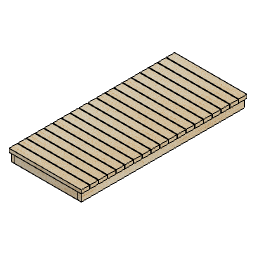
model (Autodesk Fusion 360 design; units mm, degrees)
Autodesk Fusion 360 part; units mm, degrees
sketch "Sketch1" plane through (0, 0, 0) normal (0, 0, 1) x (1, 0, 0) in component "base"
  line L0 (0, 0) -> (762, 0)
  line L1 (762, 0) -> (762, 1778)
  line L2 (762, 1778) -> (0, 1778)
  line L3 (0, 1778) -> (0, 0)
  line L4 (38.1, 38.1) -> (723.9, 38.1)
  line L5 (723.9, 38.1) -> (723.9, 1739.9)
  line L6 (723.9, 1739.9) -> (38.1, 1739.9)
  line L7 (38.1, 1739.9) -> (38.1, 38.1)
  line L8 (38.1, 1739.9) -> (38.1, 1778)
  line L9 (723.9, 1739.9) -> (723.9, 1778)
  line L10 (723.9, 38.1) -> (723.9, 0)
  line L11 (38.1, 38.1) -> (38.1, 0)
  line L12 (400.05, 1739.9) -> (361.95, 1739.9)
  line L13 (361.95, 1739.9) -> (361.95, 38.1)
  line L14 (361.95, 38.1) -> (400.05, 38.1)
  line L15 (400.05, 38.1) -> (400.05, 1739.9)
  line L16 (361.95, 889) -> (38.1, 889) construction
  line L17 (400.05, 889) -> (723.9, 889) construction
  line L18 (400.05, 1391.92) -> (723.9, 1391.92)
  line L19 (723.9, 1391.92) -> (723.9, 1430.02)
  line L20 (723.9, 1430.02) -> (400.05, 1430.02)
  line L21 (400.05, 1430.02) -> (400.05, 1391.92)
  line L22 (38.1, 386.08) -> (361.95, 386.08)
  line L23 (361.95, 386.08) -> (361.95, 347.98)
  line L24 (361.95, 347.98) -> (38.1, 347.98)
  line L25 (38.1, 347.98) -> (38.1, 386.08)
  line L26 (38.1, 1082.04) -> (361.95, 1082.04)
  line L27 (361.95, 1082.04) -> (361.95, 1043.94)
  line L28 (361.95, 1043.94) -> (38.1, 1043.94)
  line L29 (38.1, 1043.94) -> (38.1, 1082.04)
  line L30 (400.05, 734.06) -> (723.9, 734.06)
  line L31 (723.9, 734.06) -> (723.9, 695.96)
  line L32 (723.9, 695.96) -> (400.05, 695.96)
  line L33 (400.05, 695.96) -> (400.05, 734.06)
  line L34 (561.975, 734.06) -> (561.975, 889) construction
  line L35 (200.025, 386.08) -> (561.975, 695.96) construction
  line L36 (561.975, 734.06) -> (200.025, 1043.94) construction
  line L37 (561.975, 695.96) -> (561.975, 38.1) construction
  line L38 (200.025, 347.98) -> (561.975, 38.1) construction
  line L39 (200.025, 1082.04) -> (561.975, 1391.92) construction
  line L40 (200.025, 1082.04) -> (200.025, 1739.9) construction
  line L41 (561.975, 1430.02) -> (200.025, 1739.9) construction
  dimension "d3" = 1778
  dimension "d4" = 762
  dimension "d5" = -38.1
  dimension "d6" = 38.1
  dimension "d7" = 38.1
  dimension "d8" = 38.1
  dimension "d9" = 38.1
  dimension "d10" = 38.1
  constraint horizontal L0
  constraint vertical L1
  constraint horizontal L2
  constraint vertical L3
  constraint coincident L0.start L3.end
  constraint coincident L2 L8.end
  constraint perpendicular L2 L8
  constraint coincident L2 L9.end
  constraint perpendicular L2 L9
  constraint coincident L0 L10.end
  constraint perpendicular L0 L10
  constraint coincident L0 L11.end
  constraint perpendicular L0 L11
  constraint horizontal L12
  constraint vertical L13
  constraint horizontal L14
  constraint vertical L15
  constraint coincident L4 L13.end
  constraint coincident L6 L12.start
  constraint midpoint L13 L16.start
  constraint midpoint L7 L16.end
  constraint midpoint L15 L17.start
  constraint midpoint L5 L17.end
  constraint equal L16 L17
  constraint horizontal L18
  constraint vertical L19
  constraint horizontal L20
  constraint vertical L21
  constraint coincident L5 L19.end
  constraint coincident L15 L18.start
  constraint horizontal L22
  constraint vertical L23
  constraint horizontal L24
  constraint vertical L25
  constraint coincident L13 L23.end
  constraint coincident L7 L22.start
  constraint midpoint L24 L38.start
  constraint horizontal L26
  constraint vertical L27
  constraint horizontal L28
  constraint vertical L29
  constraint coincident L13 L27.end
  constraint coincident L7 L26.start
  constraint horizontal L30
  constraint vertical L31
  constraint horizontal L32
  constraint vertical L33
  constraint coincident L5 L31.end
  constraint coincident L15 L30.start
  constraint midpoint L28 L36.end
  constraint midpoint L30 L34.start
  constraint midpoint L17 L34.end
  constraint perpendicular L17 L34
  constraint midpoint L22 L35.start
  constraint midpoint L32 L35.end
  constraint equal L35 L36
  constraint coincident L4 L37.end
  constraint perpendicular L4 L37
  constraint equal L35 L38
  constraint midpoint L26 L39.start
  constraint midpoint L18 L39.end
  constraint coincident L6 L40.end
  constraint perpendicular L6 L40
  constraint equal L36 L39
  constraint midpoint L20 L41.start
  constraint equal L39 L41
  measures "d3" distance of L0.start L2.end
  measures "d4" distance of L0.start L0.end
  measures "d6" distance of L13.end L14.end
  measures "d7" distance of L22.start L24.end
  measures "d8" distance of L18.end L19.end
  measures "d9" distance of L30.end L31.end
  measures "d10" distance of L26.start L28.end
extrude "Extrude1" add sketch "Sketch1" along normal blind 88.9 contours L0 L4 L10 L11 L14 | L2 L6 L8 L9 L12 | L7 L13 L22 L23 L24 L25 | L5 L15 L30 L31 L32 L33 | L7 L13 L26 L27 L28 L29 | L5 L15 L18 L19 L20 L21 makes body 1 at (146.05, 1082.04, 29.6333) makes body 2 at (266.7, 38.1, 29.6333) makes body 3 at (508, 1391.92, 29.6333) makes body 4 at (615.95, 695.96, 29.6333) makes body 5 at (146.05, 386.08, 29.6333) makes body 6 at (495.3, 1778, 29.6333) in component "base"
extrude "Extrude2" add sketch "Sketch1" along normal blind 88.9 separate body contours L0 L2 L3 L7 L8 L11 L25 L29 | L0 L1 L2 L5 L9 L10 L19 L31 | L4 L6 L12 L13 L14 L15 L21 L23 L27 L33 makes body 7 at (361.95, 1172.6333, 29.6333) makes body 8 at (723.9, 1185.3333, 29.6333) makes body 9 at (38.1, 592.6667, 29.6333) in component "base"
sketch "Sketch1 (2)" plane through (0, 0, 88.9) normal (0, 0, 1) x (-1, 0, 0) in component "decking"
  line L0 (-38.1, 0) -> (-38.1, -1778)
  line L1 (-38.1, -1778) -> (0, -1778)
  line L2 (0, -1778) -> (0, 0)
  line L3 (0, 0) -> (-38.1, 0)
  line L4 (12.7, -1790.7) -> (-774.7, -1790.7)
  line L5 (-774.7, -1790.7) -> (-774.7, -1701.8)
  line L6 (-774.7, -1701.8) -> (12.7, -1701.8)
  line L7 (12.7, -1701.8) -> (12.7, -1790.7)
  line L8 (12.7, -1695.45) -> (-774.7, -1695.45)
  line L9 (-774.7, -1695.45) -> (-774.7, -1606.55)
  line L10 (-774.7, -1606.55) -> (12.7, -1606.55)
  line L11 (12.7, -1606.55) -> (12.7, -1695.45)
  line L12 (12.7, -1600.2) -> (-774.7, -1600.2)
  line L13 (-774.7, -1600.2) -> (-774.7, -1511.3)
  line L14 (-774.7, -1511.3) -> (12.7, -1511.3)
  line L15 (12.7, -1511.3) -> (12.7, -1600.2)
  line L16 (12.7, -1504.95) -> (-774.7, -1504.95)
  line L17 (-774.7, -1504.95) -> (-774.7, -1416.05)
  line L18 (-774.7, -1416.05) -> (12.7, -1416.05)
  line L19 (12.7, -1416.05) -> (12.7, -1504.95)
  line L20 (12.7, -1409.7) -> (-774.7, -1409.7)
  line L21 (-774.7, -1409.7) -> (-774.7, -1320.8)
  line L22 (-774.7, -1320.8) -> (12.7, -1320.8)
  line L23 (12.7, -1320.8) -> (12.7, -1409.7)
  line L24 (12.7, -1314.45) -> (-774.7, -1314.45)
  line L25 (-774.7, -1314.45) -> (-774.7, -1225.55)
  line L26 (-774.7, -1225.55) -> (12.7, -1225.55)
  line L27 (12.7, -1225.55) -> (12.7, -1314.45)
  line L28 (12.7, -1219.2) -> (-774.7, -1219.2)
  line L29 (-774.7, -1219.2) -> (-774.7, -1130.3)
  line L30 (-774.7, -1130.3) -> (12.7, -1130.3)
  line L31 (12.7, -1130.3) -> (12.7, -1219.2)
  line L32 (12.7, -1123.95) -> (-774.7, -1123.95)
  line L33 (-774.7, -1123.95) -> (-774.7, -1035.05)
  line L34 (-774.7, -1035.05) -> (12.7, -1035.05)
  line L35 (12.7, -1035.05) -> (12.7, -1123.95)
  line L36 (12.7, -1028.7) -> (-774.7, -1028.7)
  line L37 (-774.7, -1028.7) -> (-774.7, -939.8)
  line L38 (-774.7, -939.8) -> (12.7, -939.8)
  line L39 (12.7, -939.8) -> (12.7, -1028.7)
  line L40 (12.7, -933.45) -> (-774.7, -933.45)
  line L41 (-774.7, -933.45) -> (-774.7, -844.55)
  line L42 (-774.7, -844.55) -> (12.7, -844.55)
  line L43 (12.7, -844.55) -> (12.7, -933.45)
  line L44 (12.7, -838.2) -> (-774.7, -838.2)
  line L45 (-774.7, -838.2) -> (-774.7, -749.3)
  line L46 (-774.7, -749.3) -> (12.7, -749.3)
  line L47 (12.7, -749.3) -> (12.7, -838.2)
  line L48 (12.7, -742.95) -> (-774.7, -742.95)
  line L49 (-774.7, -742.95) -> (-774.7, -654.05)
  line L50 (-774.7, -654.05) -> (12.7, -654.05)
  line L51 (12.7, -654.05) -> (12.7, -742.95)
  line L52 (12.7, -647.7) -> (-774.7, -647.7)
  line L53 (-774.7, -647.7) -> (-774.7, -558.8)
  line L54 (-774.7, -558.8) -> (12.7, -558.8)
  line L55 (12.7, -558.8) -> (12.7, -647.7)
  line L56 (12.7, -552.45) -> (-774.7, -552.45)
  line L57 (-774.7, -552.45) -> (-774.7, -463.55)
  line L58 (-774.7, -463.55) -> (12.7, -463.55)
  line L59 (12.7, -463.55) -> (12.7, -552.45)
  line L60 (12.7, -457.2) -> (-774.7, -457.2)
  line L61 (-774.7, -457.2) -> (-774.7, -368.3)
  line L62 (-774.7, -368.3) -> (12.7, -368.3)
  line L63 (12.7, -368.3) -> (12.7, -457.2)
  line L64 (12.7, -361.95) -> (-774.7, -361.95)
  line L65 (-774.7, -361.95) -> (-774.7, -273.05)
  line L66 (-774.7, -273.05) -> (12.7, -273.05)
  line L67 (12.7, -273.05) -> (12.7, -361.95)
  line L68 (12.7, -266.7) -> (-774.7, -266.7)
  line L69 (-774.7, -266.7) -> (-774.7, -177.8)
  line L70 (-774.7, -177.8) -> (12.7, -177.8)
  line L71 (12.7, -177.8) -> (12.7, -266.7)
  line L72 (12.7, -171.45) -> (-774.7, -171.45)
  line L73 (-774.7, -171.45) -> (-774.7, -82.55)
  line L74 (-774.7, -82.55) -> (12.7, -82.55)
  line L75 (12.7, -82.55) -> (12.7, -171.45)
  line L76 (12.7, -76.2) -> (-774.7, -76.2)
  line L77 (-774.7, -76.2) -> (-774.7, 12.7)
  line L78 (-774.7, 12.7) -> (12.7, 12.7)
  line L79 (12.7, 12.7) -> (12.7, -76.2)
  line L80 (0, -1778) -> (12.7, -1778) construction
  line L81 (-774.7, -1778) -> (-762, -1778) construction
  line L82 (-723.9, -1778) -> (-38.1, -1778) construction
  line L83 (-381, -1778) -> (-381, -1790.7) construction
  point P0 (-762, -1778)
  dimension "d15" = 787.4
  dimension "d16" = 88.9
  dimension "d19" = 0
  dimension "d20" = 95.25
  constraint horizontal L4
  constraint vertical L5
  constraint horizontal L6
  constraint vertical L7
  constraint coincident L1.end L2.start
  constraint coincident L7 L80.end
  constraint perpendicular L7 L80
  constraint coincident L5 L81.start
  constraint coincident P0 L81.end
  constraint perpendicular L5 L81
  constraint equal L80 L81
  constraint midpoint L82 L83.start
  constraint midpoint L4 L83.end
  constraint equal L80 L83
  measures "d15" distance of L4.start L4.end
  measures "d16" distance of L4.end L5.end
extrude "Extrude1'" add sketch "Sketch1 (2)" along normal blind 38.1 separate body contours L0 L2 L3 L76 | L0 L2 L3 L76 L77 L78 L79 | L0 L2 L72 L74 | L0 L72 L73 L74 | L2 L72 L74 L75 | L0 L2 L68 L70 | L0 L68 L69 L70 | L2 L68 L70 L71 | L0 L2 L64 L66 | L0 L64 L65 L66 | L2 L64 L66 L67 | L0 L2 L60 L62 | L0 L60 L61 L62 | L2 L60 L62 L63 | L0 L2 L56 L58 | L0 L56 L57 L58 | L2 L56 L58 L59 | L0 L2 L52 L54 | L0 L52 L53 L54 | L2 L52 L54 L55 | L0 L2 L48 L50 | L0 L48 L49 L50 | L2 L48 L50 L51 | L0 L2 L44 L46 | L0 L44 L45 L46 | L2 L44 L46 L47 | L0 L2 L40 L42 | L0 L40 L41 L42 | L2 L40 L42 L43 | L0 L2 L36 L38 | L0 L36 L37 L38 | L2 L36 L38 L39 | L0 L2 L32 L34 | L0 L32 L33 L34 | L2 L32 L34 L35 | L0 L2 L28 L30 | L0 L28 L29 L30 | L2 L28 L30 L31 | L0 L2 L24 L26 | L0 L24 L25 L26 | L2 L24 L26 L27 | L0 L2 L20 L22 | L0 L20 L21 L22 | L2 L20 L22 L23 | L0 L2 L16 L18 | L0 L16 L17 L18 | L2 L16 L18 L19 | L0 L2 L12 L14 | L0 L12 L13 L14 | L2 L12 L14 L15 | L0 L2 L8 L10 | L0 L8 L9 L10 | L2 L8 L10 L11 | L0 L1 L2 L6 | L0 L1 L2 L4 L5 L6 L7 makes body 10 at (512.2333, 1540.9333, 88.9) makes body 11 at (249.7667, 1159.9333, 88.9) makes body 12 at (512.2333, 778.9333, 88.9) makes body 13 at (512.2333, 397.9333, 88.9) makes body 14 at (512.2333, 16.9333, 88.9) makes body 15 at (512.2333, 302.6833, 88.9) makes body 16 at (512.2333, 683.6833, 88.9) makes body 17 at (512.2333, 1064.6833, 88.9) makes body 18 at (512.2333, 1445.6833, 88.9) makes body 19 at (249.7667, 1636.1833, 88.9) makes body 20 at (512.2333, 1255.1833, 88.9) makes body 21 at (512.2333, 874.1833, 88.9) makes body 22 at (512.2333, 493.1833, 88.9) makes body 23 at (512.2333, 112.1833, 88.9) makes body 24 at (512.2333, 207.4333, 88.9) makes body 25 at (512.2333, 588.4333, 88.9) makes body 26 at (249.7667, 969.4333, 88.9) makes body 27 at (512.2333, 1350.4333, 88.9) makes body 28 at (512.2333, 1731.4333, 88.9) in component "decking"
component "base" placed x (1, 0, 0) y (0, 1, 0) z (0, 0, 1) at (0, 0, 0)
component "decking" placed x (1, 0, 0) y (0, 1, 0) z (0, 0, 1) at (0, 0, 0)
equation "width = 2.5 ft"
equation "length = 5'-10\""
equation "d3 = length"
equation "d4 = width"
equation "d6 = -d5"
equation "d7 = d6"
equation "d8 = d7"
equation "d9 = d8"
equation "d10 = d8"
equation "d15 = width + overhang * 2"
equation "d18 = count"
equation "overhang = 0.5 in"
equation "gap = 0.25 in"
equation "deckingCount = ceil(( length + 2 * overhang ) / 3.75 in)"
equation "count = ceil(deckingCount)"
